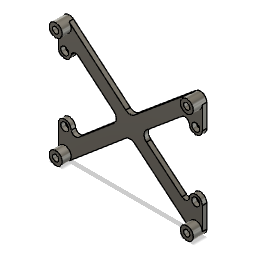
Pi3B+Bracket (Autodesk Fusion 360 design; units mm, degrees)
Autodesk Fusion 360 part; units mm, degrees
sketch "Skizze1" plane through (0, 0, 0) normal (0, 0, 1) x (1, 0, 0)
  line L0 (0, 0) -> (85, 0)
  line L1 (85, 0) -> (85, 56)
  line L2 (85, 56) -> (0, 56)
  line L3 (0, 56) -> (0, 0)
  line L4 (85, 0) -> (64, 0)
  line L5 (64, 56) -> (85, 56)
  line L6 (85, 56) -> (85, 0)
  line L7 (64, 0) -> (61.5, 0)
  line L8 (61.5, 0) -> (61.5, 3.7)
  line L9 (0, 56) -> (3.7, 56)
  line L10 (0, 52.5) -> (0, 56)
  circle A0 centre (3.5, 52.5) radius 1.375
  circle A1 centre (61.5, 52.3) radius 1.375
  circle A2 centre (61.5, 3.7) radius 1.375
  circle A3 centre (3.5, 3.5) radius 1.375
  dimension "d1" = 85
  dimension "d2" = 56
  dimension "d3" = 21
  dimension "d5" = 3.7
  dimension "d8" = 2.75
  dimension "d9" = 2.75
  dimension "d10" = 2.75
  dimension "d11" = 2.75
  dimension "d16" = 49
  dimension "d17" = 3.5
  dimension "d18" = 58
  dimension "d19" = 58
  dimension "d20" = 3.5
  dimension "d21" = 2
  dimension "d22" = 3.5
  constraint horizontal L0
  constraint vertical L1
  constraint horizontal L2
  constraint vertical L3
  constraint coincident L0.start L3.end
  constraint horizontal L4
  constraint horizontal L5
  constraint vertical L6
  constraint coincident L2 L5.start
  constraint perpendicular L0 L8
  constraint horizontal L9
  constraint vertical L10
  constraint coincident L8.end A2.centre
  measures "d1" distance of L0.start L0.end
  measures "d2" distance of L0.start L2.end
  measures "d3" distance of L0.end L4.end
  measures "d5" distance of L7.end L8.end
  measures "d8" diameter of A0
  measures "d9" diameter of A1
  measures "d10" diameter of A2
  measures "d11" diameter of A3
  measures "d16" distance of A0.centre A3.centre
  measures "d17" distance of L2 A0.centre
  measures "d18" horizontal distance of L8.end A3.centre
  measures "d19" horizontal distance of A0.centre A1.centre
  measures "d20" distance of L3 A0.centre
  measures "d22" distance of L3 A3.centre
extrude "Extrusion1" add sketch "Skizze1" along normal blind 1.3 makes body 1
fillet "Abrundung1" radius 3 4 edges at (85, 0, 0.65) (85, 56, 0.65) (0, 56, 0.65) (0, 0, 0.65) on bodies 1
sketch "Skizze2" plane through (0, 0, 1.3) normal (0, 0, 1) x (1, 0, 0)
  arc A0 (0, 3) -> (3, 0) centre (3, 3) ccw
  line L0 (3, 0) -> (82, 0)
  arc A1 (82, 0) -> (85, 3) centre (82, 3) ccw
  line L1 (85, 3) -> (85, 53)
  arc A2 (85, 53) -> (82, 56) centre (82, 53) ccw
  line L2 (82, 56) -> (3, 56)
  arc A3 (3, 56) -> (0, 53) centre (3, 53) ccw
  line L3 (0, 53) -> (0, 3)
  circle A4 centre (61.5, 52.3) radius 1.375
  circle A5 centre (61.5, 3.7) radius 1.375
  circle A6 centre (3.5, 3.5) radius 1.375
  circle A7 centre (3.5, 52.5) radius 1.375
  line L4 (65.65, 18.25) -> (87, 18.25)
  line L5 (87, 18.25) -> (87, 2.25)
  line L6 (87, 2.25) -> (65.65, 2.25)
  line L7 (65.65, 2.25) -> (65.65, 18.25)
  line L8 (69.3, 22.3) -> (87, 22.3)
  line L9 (87, 22.3) -> (87, 35.7)
  line L10 (87, 35.7) -> (69.3, 35.7)
  line L11 (69.3, 35.7) -> (69.3, 22.3)
  line L12 (69.3, 22.3) -> (87, 22.3)
  line L13 (87, 22.3) -> (87, 35.7)
  line L14 (87, 35.7) -> (69.3, 35.7)
  line L15 (69.3, 35.7) -> (69.3, 22.3)
  line L16 (87, 40.3) -> (69.3, 40.3)
  line L17 (69.3, 40.3) -> (69.3, 53.7)
  line L18 (69.3, 53.7) -> (87, 53.7)
  line L19 (87, 53.7) -> (87, 40.3)
  line L20 (7, 55.1) -> (57.8, 55.1)
  line L21 (57.8, 55.1) -> (57.8, 50.1)
  line L22 (57.8, 50.1) -> (7, 50.1)
  line L23 (7, 50.1) -> (7, 55.1)
  point P0 (7, 55.1)
  dimension "d27" = 21.35
  dimension "d28" = 16
  dimension "d31" = 17.7
  dimension "d32" = 13.4
  dimension "d33" = 17.7
  dimension "d34" = 13.4
  dimension "d36" = 17.7
  dimension "d37" = 13.4
  dimension "d44" = 50.8
  dimension "d45" = 5
  constraint horizontal L4
  constraint vertical L5
  constraint horizontal L6
  constraint vertical L7
  constraint horizontal L8
  constraint vertical L9
  constraint horizontal L10
  constraint vertical L11
  constraint horizontal L12
  constraint vertical L13
  constraint horizontal L14
  constraint vertical L15
  constraint horizontal L16
  constraint vertical L17
  constraint horizontal L18
  constraint vertical L19
  constraint horizontal L20
  constraint vertical L21
  constraint horizontal L22
  constraint vertical L23
  constraint coincident P0 L20.start
  measures "d27" distance of L4.start L4.end
  measures "d28" distance of L4.start L6.end
  measures "d31" distance of L8.start L8.end
  measures "d32" distance of L8.start L10.end
  measures "d33" distance of L8.end L8.start
  measures "d34" distance of L10.end L8.start
  measures "d36" distance of L16.start L16.end
  measures "d37" distance of L16.start L18.end
  measures "d44" distance of P0 L20.end
  measures "d45" distance of P0 L22.end
extrude "Extrusion3" add sketch "Skizze2" along normal blind 13.5 contours A1 L1 L4 L6 L7 | A1 L1 L4 L5 L6 bodies 1
extrude "Extrusion4" add sketch "Skizze2" along normal blind 16 contours L1 A2 L16 L18 L19 | L1 A2 L16 L17 L18 | L1 L8 L10 L11 L12 L14 L15 | L1 L8 L9 L10 L12 L13 L14 bodies 1
extrude "Extrusion5" add sketch "Skizze2" along normal blind 8.5 contours L20 L21 L22 L23 bodies 1
sketch "Skizze3" plane through (0, 0, 0) normal (0, 0, -1) x (-1, 0, 0)
  circle A0 centre (-61.5, 52.3) radius 1.375
  circle A1 centre (-61.5, 3.7) radius 1.375
  circle A2 centre (-3.5, 3.5) radius 1.375
  circle A3 centre (-3.5, 52.5) radius 1.375
  arc A4 (-3, 0) -> (0, 3) centre (-3, 3) ccw
  line L0 (0, 3) -> (0, 53)
  arc A5 (0, 53) -> (-3, 56) centre (-3, 53) ccw
  line L1 (-3, 56) -> (-82, 56)
  arc A6 (-82, 56) -> (-85, 53) centre (-82, 53) ccw
  line L2 (-85, 53) -> (-85, 3)
  arc A7 (-85, 3) -> (-82, 0) centre (-82, 3) ccw
  line L3 (-82, 0) -> (-3, 0)
  circle A8 centre (-61.5, 52.3) radius 1.375
  circle A9 centre (-3.5, 52.5) radius 1.375
  circle A10 centre (-3.5, 3.5) radius 1.375
  circle A11 centre (-61.5, 3.7) radius 1.375
  circle A12 centre (-3.5, 52.5) radius 2.875
  circle A13 centre (-3.5, 3.5) radius 2.875
  circle A14 centre (-61.5, 3.7) radius 2.875
  circle A15 centre (-61.5, 52.3) radius 2.875
  line L4 (-5.3585, 54.6935) -> (-32.4288, 31.7572)
  line L5 (-32.4288, 31.7572) -> (-59.6566, 54.5063)
  line L6 (-1.6415, 50.3065) -> (-27.9685, 28)
  line L7 (-36.8999, 28) -> (-63.3434, 50.0937)
  line L8 (-36.8999, 28) -> (-63.3434, 5.9063)
  line L9 (-1.6415, 5.6935) -> (-27.9685, 28)
  line L10 (-5.3585, 1.3065) -> (-32.4288, 24.2428)
  line L11 (-32.4288, 24.2428) -> (-59.6566, 1.4937)
  dimension "d49" = 1.5
  dimension "d50" = 1.5
  dimension "d51" = 1.5
  dimension "d52" = 1.5
  constraint concentric A0 A8
  constraint concentric A3 A9
  constraint concentric A2 A10
  constraint concentric A1 A11
extrude "Extrusion6" add sketch "Skizze3" along normal blind 2 separate body contours A0 A8 | A1 A11 | A2 A10 | A3 A9 | A12 | A12 A13 A14 A15 L4 L5 L6 L7 L8 L9 L10 L11 | A15 | A13 | A14 makes body 2
fillet "Abrundung2" radius 3 4 edges at (27.9685, 28, -1) (32.4288, 24.2428, -1) (36.8999, 28, -1) (32.4288, 31.7572, -1) on bodies 2
extrude "Extrusion7" add sketch "Skizze3" against normal blind 4 contours A12 | A15 | A13 | A14 bodies 2
extrude "Extrusion8" cut 4 faces at (3.0955, 3.8117, 0) (62.4164, 4.0138, 0) (61.0691, 52.7273, 0) (3.0528, 52.2418, 0) along direction (0, 0, -1) blind 5 on bodies 2 bodies 2
sketch "Skizze4" plane through (0, 0, 0) normal (0, 0, 1) x (1, 0, 0)
  arc A0 (63.3434, 5.9063) -> (59.6566, 1.4937) centre (61.5, 3.7) ccw
  line L0 (63.3434, 5.9063) -> (39.6553, 25.6978)
  arc A1 (39.6553, 30.3022) -> (39.6553, 25.6978) centre (41.5788, 28) ccw
  line L1 (39.6553, 30.3022) -> (63.3434, 50.0937)
  arc A2 (59.6566, 54.5063) -> (63.3434, 50.0937) centre (61.5, 52.3) ccw
  line L2 (59.6566, 54.5063) -> (34.3658, 33.3756)
  arc A3 (30.503, 33.389) -> (34.3658, 33.3756) centre (32.4423, 35.6778) ccw
  line L3 (30.503, 33.389) -> (5.3585, 54.6935)
  arc A4 (1.6415, 50.3065) -> (5.3585, 54.6935) centre (3.5, 52.5) ccw
  line L4 (1.6415, 50.3065) -> (25.267, 30.2889)
  arc A5 (25.267, 25.7111) -> (25.267, 30.2889) centre (23.3277, 28) ccw
  line L5 (25.267, 25.7111) -> (1.6415, 5.6935)
  arc A6 (5.3585, 1.3065) -> (1.6415, 5.6935) centre (3.5, 3.5) ccw
  line L6 (5.3585, 1.3065) -> (30.503, 22.611)
  arc A7 (34.3658, 22.6244) -> (30.503, 22.611) centre (32.4423, 20.3222) ccw
  line L7 (34.3658, 22.6244) -> (59.6566, 1.4937)
  circle A8 centre (61.5, 3.7) radius 1.375
  circle A9 centre (61.5, 52.3) radius 1.375
  circle A10 centre (3.5, 3.5) radius 1.375
  circle A11 centre (3.5, 52.5) radius 1.375
  arc A12 (30.503, 33.389) -> (34.3658, 33.3756) centre (32.4423, 35.6778) ccw
  line L8 (34.3658, 33.3756) -> (59.6566, 54.5063)
  arc A13 (39.6553, 30.3022) -> (39.6553, 25.6978) centre (41.5788, 28) ccw
  line L9 (39.6553, 25.6978) -> (63.3434, 5.9063)
  arc A14 (34.3658, 22.6244) -> (30.503, 22.611) centre (32.4423, 20.3222) ccw
  line L10 (30.503, 22.611) -> (5.3585, 1.3065)
  arc A15 (25.267, 25.7111) -> (25.267, 30.2889) centre (23.3277, 28) ccw
  line L11 (25.267, 30.2889) -> (1.6415, 50.3065)
  line L12 (59.6566, 1.4937) -> (34.3658, 22.6244)
  arc A16 (59.6566, 1.4937) -> (63.3434, 5.9063) centre (61.5, 3.7) ccw
  line L13 (63.3434, 50.0937) -> (39.6553, 30.3022)
  arc A17 (63.3434, 50.0937) -> (59.6566, 54.5063) centre (61.5, 52.3) ccw
  line L14 (5.3585, 54.6935) -> (30.503, 33.389)
  arc A18 (5.3585, 54.6935) -> (1.6415, 50.3065) centre (3.5, 52.5) ccw
  line L15 (1.6415, 5.6935) -> (25.267, 25.7111)
  arc A19 (1.6415, 5.6935) -> (5.3585, 1.3065) centre (3.5, 3.5) ccw
  line L16 (64.375, 52.3) -> (64.375, 42.3)
  line L17 (58.625, 52.3) -> (58.625, 42.3)
  circle A20 centre (61.5, 42.3) radius 1.75
  arc A21 (58.625, 42.3) -> (64.375, 42.3) centre (61.5, 42.3) ccw
  line L18 (0.625, 52.4982) -> (0.6313, 42.4982)
  line L19 (6.375, 52.4982) -> (6.3687, 42.4982)
  circle A22 centre (3.5, 42.4982) radius 1.75
  arc A23 (0.6313, 42.4982) -> (6.3687, 42.4982) centre (3.5, 42.4982) ccw
  line L20 (41.5788, 28) -> (23.3277, 28)
  line L21 (64.375, 3.7) -> (64.375, 13.7)
  line L22 (0.625, 3.5018) -> (0.6313, 13.5018)
  line L23 (58.625, 3.7) -> (58.625, 13.7)
  arc A24 (6.3687, 13.5018) -> (0.6313, 13.5018) centre (3.5, 13.5018) ccw
  circle A25 centre (3.5, 13.5018) radius 1.75
  arc A26 (64.375, 13.7) -> (58.625, 13.7) centre (61.5, 13.7) ccw
  circle A27 centre (61.5, 13.7) radius 1.75
  line L24 (6.375, 3.5018) -> (6.3687, 13.5018)
  point P0 (3.5, 3.5)
  point P1 (1.6415, 5.6935)
  point P2 (61.5, 3.7)
  point P3 (1.6415, 5.6935)
  point P4 (63.3434, 5.9063)
  point P5 (61.5, 3.7)
  point P6 (63.3434, 5.9063)
  point P7 (3.5, 3.5)
  dimension "d63" = 10
  dimension "d64" = 3.5
  dimension "d65" = 10
  dimension "d66" = 3.5
  constraint coincident A17 L16.start
  constraint vertical L16
  constraint coincident A2 L17.start
  constraint tangent A2 L17
  constraint parallel L16 L17
  constraint tangent L16 A21
  constraint concentric A20 A21
  constraint coincident A18 L18.start
  constraint concentric A22 A23
  constraint coincident A1.centre A13.centre
  constraint coincident A5.centre A15.centre
  constraint symmetric L1.end L20 P6
  constraint symmetric A2.centre L20 P5
  constraint symmetric A4.start L20 P3
  constraint symmetric A4.centre L20 P7
  constraint symmetric L16.start L20 L21.start
  constraint symmetric L16.end L20 L21.end
  constraint symmetric L17.start L20 L23.start
  constraint symmetric L17.end L20 L23.end
  constraint symmetric A20 L20 A27
  constraint symmetric A21 L20 A26
  constraint symmetric L18.start L20 L22.start
  constraint symmetric L18.end L20 L22.end
  constraint symmetric L19.start L20 L24.start
  constraint symmetric L19.end L20 A24.start
  constraint symmetric A22 L20 A25
  constraint symmetric A23 L20 A24
  measures "d63" distance of L16.start L16.end
  measures "d64" diameter of A20
  measures "d65" distance of L18.start L18.end
  measures "d66" diameter of A22
extrude "Extrusion9" add sketch "Skizze4" against normal blind 2 contours L0 L9 A16 L21 L23 A26 | L1 L13 A17 L16 L17 A21 | L5 L15 A19 L22 A24 L24 | L4 L11 A18 L18 L19 A23 bodies 2
fillet "Abrundung3" radius 2 4 edges at (6.3711, 46.2991, -1) (6.3711, 9.7009, -1) (58.625, 9.8485, -1) (58.625, 46.1515, -1) on bodies 2
copy_body "Körper->Berechn1" bodies 2 removing the originals makes body 3 in component "Halterung"
component "Halterung" placed x (1, 0, 0) y (0, 1, 0) z (0, 0, 1) at (0, 0, 0)
hidden bodies 1
named bodies: "Halterung"
